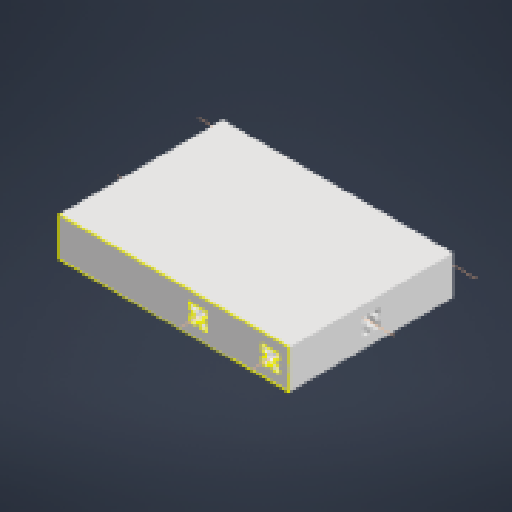
# Autodesk Inventor part: WingBox
Saved by Autodesk Inventor 2026 (Build 300175050, 175E)
## iProperties
Created: 2025-07-19
Part Number: WingBox
Material: Generic
Document SubType Name: Modeling
Designer: Cupri
Density: 1 g/cm^3
Appearance: Default
Author: Cupri
Autodesk Inventor part; units mm, degrees
ref_plane "YZ Plane" through (0, 0, 0) normal (1, 0, 0) x (0, 1, 0)
ref_plane "XZ Plane" through (0, 0, 0) normal (0, 1, 0) x (-1, 0, 0)
ref_plane "XY Plane" through (0, 0, 0) normal (0, 0, 1) x (1, 0, 0)
sketch "Sketch1" plane through (0, 0, 0) normal (0, 0, 1) x (1, 0, 0)
  line L0 (-0.011148, -7.507827) -> (0, 0)
  line L1 (0, 0) -> (20.401978, -0.030294)
  line L2 (20.401978, -0.030294) -> (20.391139, -7.329758)
  line L3 (20.391139, -7.329758) -> (16.308143, -7.323696)
  arc A0 (16.308143, -7.323696) -> (15.036259, -8.591808) centre (16.306257, -8.593694) ccw
  line L4 (15.036259, -8.591808) -> (15.032082, -11.404805)
  arc A1 (15.032082, -11.404805) -> (16.300195, -12.67669) centre (16.30208, -11.406691) ccw
  line L5 (16.300195, -12.67669) -> (20.38319, -12.682752)
  line L6 (20.38319, -12.682752) -> (20.371683, -20.432272)
  line L7 (20.371683, -20.432272) -> (12.830526, -20.421074)
  line L8 (12.830526, -20.421074) -> (12.836589, -16.338079)
  arc A2 (12.836589, -16.338079) -> (11.568476, -15.066194) centre (11.566591, -16.336193) ccw
  line L9 (11.568476, -15.066194) -> (8.755479, -15.062017)
  arc A3 (8.755479, -15.062017) -> (7.483595, -16.33013) centre (8.753594, -16.332016) ccw
  line L10 (7.483595, -16.33013) -> (7.477532, -20.413126)
  line L11 (7.477532, -20.413126) -> (-0.030294, -20.401978)
  line L12 (-0.030294, -20.401978) -> (-0.019097, -12.860821)
  line L13 (-0.019097, -12.860821) -> (4.063899, -12.866884)
  arc A4 (4.063899, -12.866884) -> (5.335783, -11.598771) centre (4.065785, -11.596885) ccw
  line L14 (5.335783, -11.598771) -> (5.33996, -8.785774)
  arc A5 (5.33996, -8.785774) -> (4.071847, -7.513889) centre (4.069962, -8.783888) ccw
  line L15 (4.071847, -7.513889) -> (-0.011148, -7.507827)
  line L16 (85.866515, -0.030871) -> (106.268493, -0.000732)
  line L17 (106.268464, -0.00081) -> (106.279555, -7.508637)
  line L18 (106.279506, -7.508596) -> (102.196511, -7.514628)
  arc A6 (102.196511, -7.514628) -> (100.928388, -8.786502) centre (102.198387, -8.784626) ccw
  line L19 (100.928388, -8.786502) -> (100.932544, -11.599499)
  arc A7 (100.932544, -11.599499) -> (102.204419, -12.867622) centre (102.202542, -11.597623) ccw
  line L20 (102.204419, -12.867622) -> (106.287414, -12.86159)
  line L21 (106.287365, -12.861631) -> (106.298505, -20.402788)
  line L22 (106.298476, -20.402759) -> (98.79065, -20.41385)
  line L23 (98.79069, -20.413801) -> (98.784659, -16.330806)
  arc A8 (98.784659, -16.330806) -> (97.512784, -15.062683) centre (97.51466, -16.332682) ccw
  line L24 (97.512784, -15.062683) -> (94.699787, -15.066839)
  arc A9 (94.699787, -15.066839) -> (93.431665, -16.338713) centre (94.701663, -16.336837) ccw
  line L25 (93.431665, -16.338713) -> (93.437696, -20.421709)
  line L26 (93.437655, -20.42166) -> (85.896499, -20.4328)
  line L27 (85.896499, -20.432272) -> (85.885051, -12.682752)
  line L28 (85.88511, -12.683267) -> (89.968105, -12.677236)
  arc A10 (89.968105, -12.677236) -> (91.236228, -11.405361) centre (89.966229, -11.407237) ccw
  line L29 (91.236228, -11.405361) -> (91.232072, -8.592364)
  arc A11 (91.232072, -8.592364) -> (89.960197, -7.324242) centre (89.962074, -8.59424) ccw
  line L30 (89.960197, -7.324242) -> (85.877202, -7.330273)
  line L31 (85.877298, -7.329758) -> (85.866515, -0.030294)
  line L32 (20.401978, -0.030294) -> (85.866515, -0.030294) construction
  line L33 (20.371683, -20.432272) -> (85.896499, -20.432272) construction
  line L34 (106.268464, -0.00081) -> (157.068464, -0.00081) construction
  line L35 (157.068464, -0.00081) -> (157.068464, -20.432272) construction
  line L36 (157.068464, -20.432272) -> (106.268464, -20.432272) construction
  line L37 (157.068464, -20.432272) -> (-142.931536, -20.432272) construction
  line L38 (-142.931536, -20.432272) -> (-142.931536, -0.00081) construction
  line L39 (-142.931536, -0.00081) -> (157.068464, -0.00081) construction
  line L40 (157.068464, -0.00081) -> (157.068464, -20.432272) construction
  line L41 (106.268464, -0.00081) -> (118.968464, -0.00081)
  line L42 (118.968464, -0.00081) -> (118.968464, -20.432272)
  line L43 (118.968464, -20.432272) -> (106.268464, -20.432272)
  line L44 (118.968464, 12.69919) -> (-142.931536, 12.69919)
  line L45 (-142.931536, 12.69919) -> (-142.931536, -33.132272) construction
  line L46 (-142.931536, -33.132272) -> (118.968464, -33.132272)
  line L47 (118.968464, -33.132272) -> (118.968464, 12.69919)
  line L48 (-142.931536, 12.69919) -> (-155.631536, 12.69919)
  line L49 (-155.631536, 12.69919) -> (-155.631536, -33.132272)
  line L50 (-155.631536, -33.132272) -> (-142.931536, -33.132272)
  line L51 (-142.931536, -33.132272) -> (-142.931536, 12.69919)
  point P0 (0, 0)
  point P1 (15.036259, -8.591808)
  point P2 (16.300195, -12.67669)
  point P3 (11.568476, -15.066194)
  point P4 (7.483595, -16.33013)
  point P5 (-0.030294, -20.401978)
  point P6 (5.335783, -11.598771)
  point P7 (4.071847, -7.513889)
  point P8 (106.268464, -0.000732)
  point P9 (106.279555, -7.508596)
  point P10 (100.928388, -8.786502)
  point P11 (106.287365, -12.86159)
  point P12 (106.298505, -20.402759)
  point P13 (98.79069, -20.41385)
  point P14 (97.512784, -15.062683)
  point P15 (93.437696, -20.42166)
  point P16 (85.896499, -20.4328)
  point P17 (85.885051, -12.683267)
  point P18 (91.236228, -11.405361)
  point P19 (85.877299, -7.330273)
  point P20 (85.866516, -0.030871)
  dimension "d0" = 50.8
  dimension "d1" = 300
  dimension "d2" = 12.7
  dimension "d3" = 12.7
  dimension "d4" = 12.7
  dimension "d5" = 12.7
  constraints: 104 end point, 36 parallel, 24 point on circle, 24 tangent, 12 centre point, 11 equal radius, 7 perpendicular, 6 horizontal, 3 point on line
  measures "d0" distance of L35.end L36.end
  measures "d1" distance of L38.end L39.end
  measures "d2" distance of L42.end L43.end
  measures "d3" distance between parallel lines of L39 L44
  measures "d4" distance between parallel lines of L46 L37
  measures "d5" distance of L50.end L49.end
extrude "Extrusion1" add sketch "Sketch1" along normal blind 195
sketch "Sketch2" plane through (0, 0, 195) normal (0, 0, 1) x (1, 0, 0)
  line L0 (-155.631536, 12.69919) -> (-155.631536, -33.132272)
  line L1 (-155.631536, -33.132272) -> (118.968464, -33.132272)
  line L2 (118.968464, -33.132272) -> (118.968464, 12.69919)
  line L3 (118.968464, 12.69919) -> (-155.631536, 12.69919)
  line L4 (-0.011148, -7.507827) -> (0, 0)
  line L5 (0, 0) -> (20.401978, -0.030294)
  line L6 (20.401978, -0.030294) -> (20.391139, -7.329758)
  line L7 (20.391139, -7.329758) -> (16.308143, -7.323696)
  arc A0 (16.308143, -7.323696) -> (15.036259, -8.591808) centre (16.306257, -8.593694) ccw
  line L8 (15.036259, -8.591808) -> (15.032082, -11.404805)
  arc A1 (15.032082, -11.404805) -> (16.300195, -12.67669) centre (16.30208, -11.406691) ccw
  line L9 (16.300195, -12.67669) -> (20.38319, -12.682752)
  line L10 (20.38319, -12.682752) -> (20.371683, -20.432272)
  line L11 (20.371683, -20.432272) -> (12.830526, -20.421074)
  line L12 (12.830526, -20.421074) -> (12.836589, -16.338079)
  arc A2 (12.836589, -16.338079) -> (11.568476, -15.066194) centre (11.566591, -16.336193) ccw
  line L13 (11.568476, -15.066194) -> (8.755479, -15.062017)
  arc A3 (8.755479, -15.062017) -> (7.483595, -16.33013) centre (8.753594, -16.332016) ccw
  line L14 (7.483595, -16.33013) -> (7.477532, -20.413126)
  line L15 (7.477532, -20.413126) -> (-0.030294, -20.401978)
  line L16 (-0.030294, -20.401978) -> (-0.019097, -12.860821)
  line L17 (-0.019097, -12.860821) -> (4.063899, -12.866884)
  arc A4 (4.063899, -12.866884) -> (5.335783, -11.598771) centre (4.065785, -11.596885) ccw
  line L18 (5.335783, -11.598771) -> (5.33996, -8.785774)
  arc A5 (5.33996, -8.785774) -> (4.071847, -7.513889) centre (4.069962, -8.783888) ccw
  line L19 (4.071847, -7.513889) -> (-0.011148, -7.507827)
  arc A6 (100.932544, -11.599499) -> (102.204419, -12.867622) centre (102.202542, -11.597623) ccw
  line L20 (102.204419, -12.867622) -> (106.287365, -12.86159)
  line L21 (106.287365, -12.86159) -> (106.298505, -20.402759)
  line L22 (106.298505, -20.402759) -> (98.79069, -20.41385)
  line L23 (98.79069, -20.41385) -> (98.784659, -16.330806)
  arc A7 (98.784659, -16.330806) -> (97.512784, -15.062683) centre (97.51466, -16.332682) ccw
  line L24 (97.512784, -15.062683) -> (94.699787, -15.066839)
  arc A8 (94.699787, -15.066839) -> (93.431665, -16.338713) centre (94.701663, -16.336837) ccw
  line L25 (93.431665, -16.338713) -> (93.437696, -20.42166)
  line L26 (93.437696, -20.42166) -> (85.896499, -20.4328)
  line L27 (85.896499, -20.4328) -> (85.885051, -12.683267)
  line L28 (85.885051, -12.683267) -> (89.968105, -12.677236)
  arc A9 (89.968105, -12.677236) -> (91.236228, -11.405361) centre (89.966229, -11.407237) ccw
  line L29 (91.236228, -11.405361) -> (91.232072, -8.592364)
  arc A10 (91.232072, -8.592364) -> (89.960197, -7.324242) centre (89.962074, -8.59424) ccw
  line L30 (89.960197, -7.324242) -> (85.877299, -7.330273)
  line L31 (85.877299, -7.330273) -> (85.866516, -0.030871)
  line L32 (85.866516, -0.030871) -> (106.268464, -0.000732)
  line L33 (106.268464, -0.000732) -> (106.279555, -7.508596)
  line L34 (106.279555, -7.508596) -> (102.196511, -7.514628)
  arc A11 (102.196511, -7.514628) -> (100.928388, -8.786502) centre (102.198387, -8.784626) ccw
  line L35 (100.928388, -8.786502) -> (100.932544, -11.599499)
  line L36 (0, 0) -> (20.371683, -20.432272) construction
  line L37 (20.401978, -0.030294) -> (-0.030294, -20.401978) construction
  line L38 (85.866516, -0.030871) -> (106.298507, -20.402759) construction
  line L39 (85.896499, -20.4328) -> (106.268464, -0.000732) construction
  point P0 (0, 0)
  point P1 (10.185842, -10.216136)
  point P2 (96.082482, -10.216766)
  constraints: 8 end point, 2 midpoint, 2 perpendicular, 1 point on line
sketch "Sketch3" plane through (-155.631536, -33.132272, 0) normal (-1, 0, 0) x (0, 0, 1)
  line L0 (87.303023, 25.62401) -> (87.314171, 33.131836)
  line L1 (87.314171, 33.131836) -> (107.716148, 33.101542)
  line L2 (107.716148, 33.101542) -> (107.705309, 25.802078)
  line L3 (107.705309, 25.802078) -> (103.622314, 25.808141)
  arc A0 (103.622314, 25.808141) -> (102.35043, 24.540028) centre (103.620428, 24.538142) ccw
  line L4 (102.35043, 24.540028) -> (102.346253, 21.727031)
  arc A1 (102.346253, 21.727031) -> (103.614365, 20.455146) centre (103.616251, 21.725145) ccw
  line L5 (103.614365, 20.455146) -> (107.697361, 20.449084)
  line L6 (107.697361, 20.449084) -> (107.685854, 12.699564)
  line L7 (107.685854, 12.699564) -> (100.144697, 12.710762)
  line L8 (100.144697, 12.710762) -> (100.15076, 16.793757)
  arc A2 (100.15076, 16.793757) -> (98.882647, 18.065642) centre (98.880761, 16.795643) ccw
  line L9 (98.882647, 18.065642) -> (96.06965, 18.069819)
  arc A3 (96.06965, 18.069819) -> (94.797766, 16.801706) centre (96.067764, 16.79982) ccw
  line L10 (94.797766, 16.801706) -> (94.791703, 12.718711)
  line L11 (94.791703, 12.718711) -> (87.283876, 12.729859)
  line L12 (87.283876, 12.729859) -> (87.295074, 20.271015)
  line L13 (87.295074, 20.271015) -> (91.37807, 20.264953)
  arc A4 (91.37807, 20.264953) -> (92.649954, 21.533065) centre (91.379955, 21.534951) ccw
  line L14 (92.649954, 21.533065) -> (92.654131, 24.346062)
  arc A5 (92.654131, 24.346062) -> (91.386018, 25.617947) centre (91.384132, 24.347948) ccw
  line L15 (91.386018, 25.617947) -> (87.303023, 25.62401)
  line L16 (0, 45.831462) -> (0, 0)
  line L17 (0, 0) -> (195, 0)
  line L18 (195, 45.831462) -> (195, 0)
  line L19 (0, 45.831462) -> (195, 45.831462)
  line L20 (0, 45.831462) -> (195, 0) construction
  line L21 (195, 45.831462) -> (0, 0) construction
  line L22 (87.314171, 33.131836) -> (107.685854, 12.699564) construction
  line L23 (87.283876, 12.729859) -> (107.716148, 33.101542) construction
  point P0 (0, 33.132272)
  point P1 (87.314171, 33.131836)
  point P2 (97.500012, 22.9157)
  constraints: 40 end point, 12 point on circle, 6 centre point, 1 midpoint, 1 perpendicular
extrude "Extrusion2" cut sketch "Sketch3" against normal blind 302.949991 contours L0 L1 L2 L3 A0 L4 A1 L5 L6 L7 L8 A2 L9 A3 L10 L11 L12 L13 A4 L14 A5 L15
sketch "Sketch4" plane through (-155.631536, -33.132272, 0) normal (-1, 0, 0) x (0, 0, 1)
  line L0 (107.716148, 33.101542) -> (87.314171, 33.131836)
  line L1 (100.144697, 12.710762) -> (107.685854, 12.699564)
  line L2 (87.314171, 33.131836) -> (107.685854, 12.699564) construction
  line L3 (0, 12.699472) -> (195, 12.699472)
  line L4 (87.355668, 12.699472) -> (107.685854, 33.101587) construction
  point P0 (0, 33.132272)
  point P1 (97.520761, 22.900529)
  constraints: 4 end point, 2 point on line, 1 midpoint
sketch "Sketch5" plane through (0, 0, 0) normal (0, 0, -1) x (-1, 0, 0)
  line L0 (-106.268509, -0.03073) -> (-106.279292, -7.330194)
  line L1 (-106.268509, -0.03073) -> (-45.768509, -0.03073)
  line L2 (-45.768509, -0.03073) -> (-45.768509, 4.46927)
  line L3 (-45.768509, 4.46927) -> (-106.268509, 4.46927)
  line L4 (-106.268509, 4.46927) -> (-106.268509, -0.03073) construction
  line L5 (-106.268509, -0.03073) -> (-118.968464, -0.03073)
  line L6 (-106.268509, 4.46927) -> (-107.268509, 4.46927)
  line L7 (-107.268509, 4.46927) -> (-107.268509, -0.03073)
  line L8 (-107.268509, -0.03073) -> (-106.268509, -0.03073)
  line L9 (-106.268509, -0.03073) -> (-106.268509, 4.46927) construction
  line L10 (0, 0) -> (-20.401978, -0.030294)
  line L11 (-20.401978, -0.030294) -> (40.098022, -0.030294)
  line L12 (40.098022, -0.030294) -> (40.098022, 4.469706)
  line L13 (40.098022, 4.469706) -> (-20.401978, 4.469706)
  line L14 (-20.401978, 4.469706) -> (-20.401978, -0.030294) construction
  line L15 (-20.401977, -0.03073) -> (-85.961962, -0.03073)
  line L16 (-20.401978, 4.469706) -> (-21.401978, 4.469706)
  line L17 (-21.401978, 4.469706) -> (-21.401978, -0.03073)
  line L18 (-21.401978, -0.03073) -> (-20.401978, -0.03073)
  line L19 (-20.401978, -0.03073) -> (-20.401978, 4.469706) construction
  line L20 (-21.401978, 4.469706) -> (40.098022, 4.469706)
  line L21 (40.098022, 4.469706) -> (40.098022, -0.030294)
  line L22 (40.098022, -0.030294) -> (-21.401978, -0.030294)
  line L23 (-21.401978, -0.030294) -> (-21.401978, 4.469706)
  dimension "d10" = 4.5
  dimension "d11" = 60.5
  dimension "d12" = 1
  dimension "d13" = 60.5
  dimension "d14" = 4.5
  dimension "d15" = 1
  constraints: 40 end point, 10 parallel, 5 horizontal, 5 perpendicular, 2 point on line
  measures "d10" distance of L3.end L0.start
  measures "d11" distance of L2.end L3.end
  measures "d12" distance of L8.end L7.end
  measures "d13" distance of L13.end L12.end
  measures "d14" distance of L13.end L10.end
  measures "d15" distance of L18.end L17.end
extrude "Extrusion3" cut sketch "Sketch5" against normal blind 302.949991
sketch "Sketch7" plane through (-155.631536, -33.132272, 0) normal (-1, 0, 0) x (0, 0, 1)
  line L0 (0, 12.719146) -> (94.498272, 12.719146)
  line L1 (67.520761, 12.719146) -> (127.520761, 12.719146)
  line L2 (127.520761, 12.719146) -> (127.520761, 8.219146)
  line L3 (127.520761, 8.219146) -> (67.520761, 8.219146)
  line L4 (67.520761, 8.219146) -> (67.520761, 12.719146)
  line L5 (67.520761, 12.719146) -> (127.520761, 12.719146)
  line L6 (127.520761, 12.719146) -> (127.520761, 13.719146)
  line L7 (127.520761, 13.719146) -> (67.520761, 13.719146)
  line L8 (67.520761, 13.719146) -> (67.520761, 12.719146)
  point P0 (0, 33.132272)
  point P1 (97.520761, 22.900529)
  dimension "d18" = 60
  dimension "d19" = 30
  dimension "d20" = 4.5
  dimension "d23" = 1
  constraints: 16 end point, 4 parallel, 2 horizontal, 2 perpendicular, 1 point on line
  measures "d18" distance of L2.end L3.end
  measures "d19" distance from line of point (97.521, 22.901) L4
  measures "d20" distance between parallel lines of L1 L3
  measures "d23" distance of L5.end L6.end
extrude "Extrusion4" cut sketch "Sketch7" against normal blind 76.2
body "Solid1"
